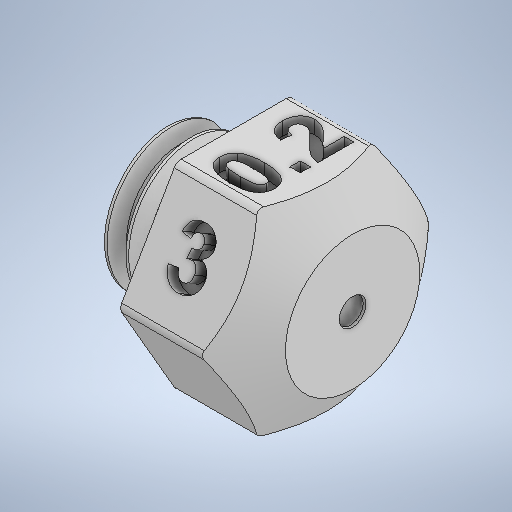
# Autodesk Inventor part: Part1
Saved by Autodesk Inventor 2025.2 (Build 292293000, 293)
## iProperties
Created: 2026-03-09
Part Number: Part1
Material: Generic
Document SubType Name: Modeling
Designer: Simon
Density: 1 g/cm^3
Appearance: Default
Author: Simon
Autodesk Inventor part; units mm, degrees
ref_plane "YZ Plane" through (0, 0, 0) normal (1, 0, 0) x (0, 1, 0)
ref_plane "XZ Plane" through (0, 0, 0) normal (0, 1, 0) x (-1, 0, 0)
ref_plane "XY Plane" through (0, 0, 0) normal (0, 0, 1) x (1, 0, 0)
sketch "Sketch1" plane through (0, 0, 0) normal (0, 0, 1) x (1, 0, 0)
  line L0 (0, 0) -> (0, 1.25)
  line L1 (0, 1.25) -> (50, 1.25)
  line L2 (0, 0) -> (0, 0.4751)
  line L3 (0, 0.4751) -> (50, 0.4751)
  line L4 (0, 0) -> (0, 0.4969)
  line L5 (0, 0.4969) -> (50, 0.4969)
  line L6 (0, 0) -> (0, 2.5)
  line L7 (0, 2.5) -> (2.5, 2.5)
  line L8 (2.5, 2.5) -> (2.5, 1.25)
  line L9 (2.5, 1.25) -> (2.5, 4.25)
  line L10 (2.5, 1.25) -> (6.7109, 1.25) construction
  line L11 (2.5, 4.25) -> (5.5, 4.25)
  line L12 (5.5, 4.25) -> (5.5, 1.25)
  line L13 (5.5, 1.25) -> (6.8421, 0.4751)
  line L14 (5.5, 1.25) -> (9.25, 1.25) construction
  line L15 (6.8421, 0.4751) -> (6.9232, 0.4969)
  line L16 (6.8421, 0.4751) -> (6.926, 0.4751) construction
  line L17 (6.9232, 0.4969) -> (6.9232, 2.4969)
  line L18 (6.9232, 2.4969) -> (5.5, 4.25)
  line L19 (0, 0) -> (50, 0)
  dimension "d0" = 1.25
  dimension "d1" = 50
  dimension "d2" = 0.4751
  dimension "d3" = 0.4969
  dimension "d4" = 2.5
  dimension "d5" = 2.5
  dimension "d6" = 3
  dimension "d8" = 3
  dimension "d9" = 30
  dimension "d10" = 15
  dimension "d12" = 2
  dimension "d13" = 50
  constraints: 40 end point, 7 perpendicular, 7 point on line, 5 horizontal, 2 vertical, 1 equal length
  measures "d0" distance of L0.start L0.end
  measures "d1" distance of L0.end L1.end
  measures "d2" distance of L0.start L2.end
  measures "d3" distance of L0.start L4.end
  measures "d4" distance of L0.start L6.end
  measures "d5" distance of L6.end L7.end
  measures "d6" distance of L8.end L9.end
  measures "d8" distance of L9.end L11.end
  measures "d9" angle of L13 L14
  measures "d10" angle of L16 L15
  measures "d12" distance of L15.end L17.end
  measures "d13" distance of L0.start L19.end
revolve "Revolution1" add sketch "Sketch1" angle 360 about axis through (0, 0, 0) along (1, 0, 0) contours L13 L5 L15 | L6 L7 L8 L1 | L13 L1 L17 L5 | L8 L9 L11 L12 L1 | L12 L18 L17 L1
sketch "Sketch2" plane through (2.5, 0, 0) normal (-1, 0, 0) x (0, 0, 1)
  circle A0 centre (0, 0) radius 4.25 projected
  line L0 (-4.25, 0) -> (4.25, 0)
  circle A1 centre (0, 0) radius 0.4751 projected
  line L1 (4.25, 0) -> (2.125, -3.6806)
  line L2 (2.125, -3.6806) -> (-2.125, -3.6806)
  line L3 (-2.125, -3.6806) -> (-4.25, 0)
  line L4 (-4.25, 0) -> (-2.125, 3.6806)
  line L5 (-2.125, 3.6806) -> (2.125, 3.6806)
  line L6 (2.125, 3.6806) -> (4.25, 0)
  circle A2 centre (0, 0) radius 1.25
  constraints: 14 end point, 2 coincident, 2 point on circle, 1 centre point, 1 horizontal, 13 other
extrude "Extrusion1" cut sketch "Sketch2" against normal through all contours L6 A0 | A0 L1 | L5 A0 | A0 L2 | L4 A0 | A0 L3
fillet "Fillet1" radius 0.3 6 edges at (4, 3.6806, 2.125) (4, 3.6806, -2.125) (4, 0, -4.25) (4, -3.6806, -2.125) (4, -3.6806, 2.125) (4, 0, 4.25)
sketch "Sketch3" plane through (0, 0, 0) normal (0, 0, 1) x (1, 0, 0)
  line L0 (-0.35, 1.8938) -> (0.45, 1.8938)
  line L1 (-0.35, 1.8938) -> (0.05, 2.5866)
  line L2 (-0.35, 1.8938) -> (0.45, 1.8938) construction
  line L3 (0.05, 2.5866) -> (0.45, 1.8938)
  line L4 (-0.0972, 3.8266) -> (0.7028, 3.8266) construction
  line L5 (0.05, 2.5866) -> (0.05, 1.8938)
  line L6 (0.05, 1.8938) -> (0.05, 2.0671)
  line L7 (0.05, 2.0671) -> (0.45, 2.0671)
  line L8 (0.45, 2.0671) -> (-0.35, 2.0671)
  line L9 (0.05, 2.5866) -> (0.05, 2.5)
  line L10 (0.05, 2.5) -> (0.45, 2.5)
  line L11 (0.45, 2.5) -> (-0.35, 2.5)
  line L12 (-0.35, 1.8938) -> (-1.15, 1.8938)
  line L13 (0.05, 2.5866) -> (-0.75, 2.5866)
  line L14 (-0.75, 2.5866) -> (-1.15, 1.8938)
  line L15 (-0.35, 1.8938) -> (-0.75, 2.5866)
  line L16 (-0.35, 2.0671) -> (-1.15, 2.0671)
  line L17 (-0.35, 2.5) -> (-0.8, 2.5)
  line L18 (-0.75, 2.5866) -> (-0.75, 1.8938)
  line L19 (-0.35, 1.8938) -> (-0.35, 1.9938)
  circle A0 centre (-0.35, 2.0938) radius 0.1
  line L20 (-0.4077, 1.9938) -> (-0.2923, 1.9938)
  line L21 (0, 2.5) -> (2.5, 2.5) projected
  line L22 (0, 2.5) -> (-0.7, 2.5)
  line L23 (-0.7, 2.5) -> (-0.4366, 2.0438)
  line L24 (-0.4366, 2.0438) -> (-0.2634, 2.0438)
  line L25 (-0.2634, 2.0438) -> (0, 2.5)
  circle A1 centre (-0.35, 2.0938) radius 0.1
  point P0 (0, 0)
  point P1 (0, 2.5)
  dimension "d18" = 0.8
  dimension "d19" = 60
  dimension "d20" = 60
  dimension "d21" = 0.1732
  dimension "d22" = 0.0866
  dimension "d23" = 0.8
  dimension "d24" = 0.1
  dimension "d25" = 0.8
  constraints: 50 end point, 13 point on line, 7 horizontal, 4 tangent, 3 midpoint, 2 centre point, 2 equal length, 2 perpendicular, 2 point on circle, 1 coincident, 1 collinear, 1 concentric, 1 parallel, 1 vertical
  measures "d18" distance of L2.start L0.end
  measures "d19" angle of L2 L1
  measures "d20" angle of L3 L4
  measures "d21" distance of L6.start L7.start
  measures "d22" distance of L3.start L10.start
  measures "d23" distance of L2.start L12.end
  measures "d24" distance of L2.start L19.end
  measures "d25" distance between parallel lines of L5 L18
coil "Coil1" sketch "Sketch3" operation cut axis through (-10, 0, 0) along (1, 0, 0) pitch 0.8 turns 4 hand right contours A0 L24 | L24 L15 L16 L8 L1 | A0 L15 L17 L11 L1 | L8 L16 A0
extrude "Extrusion2" add sketch "Sketch2" against normal blind 3 contours L1 L2 L3 L0 A2 | L0 A2 L4 L5 L6
fillet "Fillet2" radius 0.3 6 edges at (4, 3.6806, -2.125) (4, 3.6806, 2.125) (4, 0, 4.25) (4, -3.6806, 2.125) (4, -3.6806, -2.125) (4, 0, -4.25)
sketch "Sketch4" plane through (2.5, 3.6806, 1.9518) normal (0, 1, 0) x (1, 0, 0)
  line L0 (0.6481, 0.021) -> (0.6481, 3.9037) construction
  line L1 (0.6481, 3.9037) -> (2.6893, 3.9037) construction
  line L2 (2.6893, 3.9037) -> (2.6893, 0.021) construction
  line L3 (2.6893, 0.021) -> (0.6481, 0.021) construction
  spline S0 degree 2 poles (0.6481, 0.7878) (0.6481, 1.079) (0.8555, 1.2421) knots 0 0 0 1 1 1
  spline S1 degree 2 poles (0.8555, 1.2421) (1.1009, 1.4372) (1.6695, 1.4372) knots 0 0 0 1 1 1
  spline S2 degree 2 poles (1.6695, 1.4372) (2.2366, 1.4372) (2.485, 1.2406) knots 0 0 0 1 1 1
  spline S3 degree 2 poles (2.485, 1.2406) (2.6893, 1.079) (2.6893, 0.7878) knots 0 0 0 1 1 1
  spline S4 degree 2 poles (2.6893, 0.7878) (2.6893, 0.4951) (2.2411, 0.1384) (1.6649, 0.1384) knots 0 0 0 1 2 2 2
  spline S5 degree 2 poles (1.6649, 0.1384) (1.1009, 0.1384) (0.8524, 0.3351) knots 0 0 0 1 1 1
  spline S6 degree 2 poles (0.8524, 0.3351) (0.6481, 0.4967) (0.6481, 0.7878) knots 0 0 0 1 1 1
  spline S7 degree 2 poles (0.9667, 0.7878) (0.9667, 0.7177) (1.0552, 0.6095) (1.1695, 0.579) knots 0 0 0 1 2 2 2
  spline S8 degree 2 poles (1.1695, 0.579) (1.3174, 0.5393) (1.6695, 0.5393) knots 0 0 0 1 1 1
  spline S9 degree 2 poles (1.6695, 0.5393) (2.0201, 0.5393) (2.2838, 0.611) (2.3707, 0.7177) (2.3707, 0.7878) knots 0 0 0 1 2 3 3 3
  spline S10 degree 2 poles (2.3707, 0.7878) (2.3707, 0.8579) (2.2823, 0.9662) (2.168, 0.9967) knots 0 0 0 1 2 2 2
  spline S11 degree 2 poles (2.168, 0.9967) (2.0201, 1.0363) (1.6695, 1.0363) knots 0 0 0 1 1 1
  spline S12 degree 2 poles (1.6695, 1.0363) (1.3174, 1.0363) (1.0552, 0.9646) (0.9667, 0.8579) (0.9667, 0.7878) knots 0 0 0 1 2 3 3 3
  line L4 (2.6558, 1.7741) -> (2.2716, 1.7741)
  line L5 (2.2716, 1.7741) -> (2.2716, 2.1582)
  line L6 (2.2716, 2.1582) -> (2.6558, 2.1582)
  line L7 (2.6558, 2.1582) -> (2.6558, 1.7741)
  line L8 (2.2991, 3.7634) -> (2.6558, 3.7634)
  line L9 (2.6558, 3.7634) -> (2.6558, 2.4204)
  spline S13 degree 2 poles (2.6558, 2.4204) (2.4545, 2.4418) (2.0933, 2.6598) (1.7945, 2.9829) knots 0 0 0 1 2 2 2
  spline S14 degree 2 poles (1.7945, 2.9829) (1.5536, 3.2421) (1.4667, 3.3) knots 0 0 0 1 1 1
  spline S15 degree 2 poles (1.4667, 3.3) (1.3478, 3.3793) (1.232, 3.3793) knots 0 0 0 1 1 1
  spline S16 degree 2 poles (1.232, 3.3793) (1.1039, 3.3793) (0.9667, 3.2421) (0.9667, 3.1201) knots 0 0 0 1 2 2 2
  spline S17 degree 2 poles (0.9667, 3.1201) (0.9667, 3.0012) (1.1116, 2.8595) (1.2792, 2.8488) knots 0 0 0 1 2 2 2
  line L10 (1.2792, 2.8488) -> (1.2411, 2.4662)
  spline S18 degree 2 poles (1.2411, 2.4662) (0.9241, 2.4997) (0.6481, 2.8595) (0.6481, 3.1293) knots 0 0 0 1 2 2 2
  spline S19 degree 2 poles (0.6481, 3.1293) (0.6481, 3.425) (0.9667, 3.7634) (1.2045, 3.7634) knots 0 0 0 1 2 2 2
  spline S20 degree 2 poles (1.2045, 3.7634) (1.3387, 3.7634) (1.5826, 3.6674) (1.7167, 3.5622) knots 0 0 0 1 2 2 2
  spline S21 degree 2 poles (1.7167, 3.5622) (1.8052, 3.4921) (2.1375, 3.1293) (2.2472, 3.0317) (2.2991, 3.0028) knots 0 0 0 1 2 3 3 3
  line L11 (2.2991, 3.0028) -> (2.2991, 3.7634)
  point P0 (-2.5, 1.9518)
  constraints: 2 other
extrude "Extrusion3" cut sketch "Sketch4" against normal blind 0.5
sketch "Sketch5" plane through (2.5, 0.15, 4.1634) normal (0, 0.5, 0.866) x (1, 0, 0)
  line L0 (0.8475, 3.04) -> (2.4008, 3.04) construction
  line L1 (2.4008, 3.04) -> (2.4008, 1.0324) construction
  line L2 (2.4008, 1.0324) -> (0.8475, 1.0324) construction
  line L3 (0.8475, 1.0324) -> (0.8475, 3.04) construction
  line L4 (0.9527, 1.5644) -> (1.3231, 1.6102)
  spline S0 degree 2 poles (1.3231, 1.6102) (1.3414, 1.4684) (1.4969, 1.3175) (1.6066, 1.3175) knots 0 0 0 1 2 2 2
  spline S1 degree 2 poles (1.6066, 1.3175) (1.7255, 1.3175) (1.8871, 1.4974) (1.8871, 1.6498) knots 0 0 0 1 2 2 2
  spline S2 degree 2 poles (1.8871, 1.6498) (1.8871, 1.7946) (1.7332, 1.9638) (1.6219, 1.9638) knots 0 0 0 1 2 2 2
  spline S3 degree 2 poles (1.6219, 1.9638) (1.5487, 1.9638) (1.4466, 1.9349) knots 0 0 0 1 1 1
  line L5 (1.4466, 1.9349) -> (1.4893, 2.2474)
  spline S4 degree 2 poles (1.4893, 2.2474) (1.6447, 2.2428) (1.8079, 2.3861) (1.8079, 2.505) knots 0 0 0 1 2 2 2
  spline S5 degree 2 poles (1.8079, 2.505) (1.8079, 2.6056) (1.6874, 2.7245) (1.5883, 2.7245) knots 0 0 0 1 2 2 2
  spline S6 degree 2 poles (1.5883, 2.7245) (1.4893, 2.7245) (1.3505, 2.5888) (1.3353, 2.4577) knots 0 0 0 1 2 2 2
  line L6 (1.3353, 2.4577) -> (0.9816, 2.5172)
  spline S7 degree 2 poles (0.9816, 2.5172) (1.0182, 2.6986) (1.1676, 2.9166) (1.4329, 3.04) (1.599, 3.04) knots 0 0 0 1 2 3 3 3
  spline S8 degree 2 poles (1.599, 3.04) (1.881, 3.04) (2.0518, 2.8602) knots 0 0 0 1 1 1
  spline S9 degree 2 poles (2.0518, 2.8602) (2.192, 2.7138) (2.192, 2.5278) knots 0 0 0 1 1 1
  spline S10 degree 2 poles (2.192, 2.5278) (2.192, 2.2656) (1.9039, 2.1086) knots 0 0 0 1 1 1
  spline S11 degree 2 poles (1.9039, 2.1086) (2.0761, 2.072) (2.2804, 1.8144) (2.2804, 1.633) knots 0 0 0 1 2 2 2
  spline S12 degree 2 poles (2.2804, 1.633) (2.2804, 1.3693) (1.8963, 0.9989) (1.6097, 0.9989) knots 0 0 0 1 2 2 2
  spline S13 degree 2 poles (1.6097, 0.9989) (1.3383, 0.9989) (0.9816, 1.3114) (0.9527, 1.5644) knots 0 0 0 1 2 2 2
  point P0 (-2.5, 1.9518)
  constraints: 2 other
extrude "Extrusion4" cut sketch "Sketch5" against normal blind 0.5
body "Solid1"
